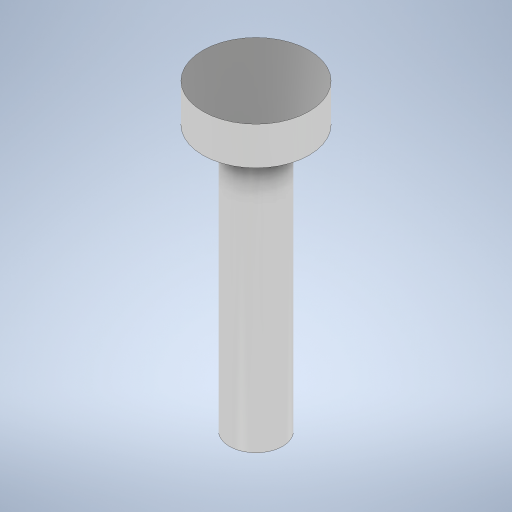
# Autodesk Inventor part: tornillo_7_21
Saved by Autodesk Inventor 2024 (Build 280153000, 153)
## iProperties
Created: 2023-05-06
Part Number: tornillo_7_21
Material: Generic
Document SubType Name: Modeling
Designer: Diego
Density: 1 g/cm^3
Appearance: Default
Author: Diego
Autodesk Inventor part; units mm, degrees
ref_plane "YZ Plane" through (0, 0, 0) normal (1, 0, 0) x (0, 1, 0)
ref_plane "XZ Plane" through (0, 0, 0) normal (0, 1, 0) x (-1, 0, 0)
ref_plane "XY Plane" through (0, 0, 0) normal (0, 0, 1) x (1, 0, 0)
sketch "Sketch1" plane through (0, 0, 0) normal (0, 1, 0) x (-1, 0, 0)
  circle A0 centre (0, 0) radius 3.5
  dimension "d0" = 7
  constraints: 1 centre point, 1 coincident
  measures "d0" diameter of A0
extrude "Extrusion1" add sketch "Sketch1" along normal blind 2.5
sketch "Sketch2" plane through (0, 0, 0) normal (0, -1, 0) x (1, 0, 0)
  circle A0 centre (0, 0) radius 1.75
  dimension "d3" = 3.5
  constraints: 1 centre point, 1 coincident
  measures "d3" diameter of A0
extrude "Extrusion2" add sketch "Sketch2" along normal blind 17.5
body "Solid1"
